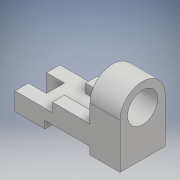
# Autodesk Inventor part: трон
Saved by Autodesk Inventor 2018 (Build 220112000, 112)
## iProperties
Created: 2020-04-15
Part Number: трон
Material: Типовые
Document SubType Name: Modeling
Designer: 2000
Density: 1 g/cm^3
Appearance: По умолчанию
Author: 2000
Autodesk Inventor part; units mm, degrees
ref_plane "YZ Plane" through (0, 0, 0) normal (1, 0, 0) x (0, 1, 0)
ref_plane "XZ Plane" through (0, 0, 0) normal (0, 1, 0) x (-1, 0, 0)
ref_plane "XY Plane" through (0, 0, 0) normal (0, 0, 1) x (1, 0, 0)
sketch "Эскиз1" plane through (0, 0, 0) normal (0, 0, 1) x (1, 0, 0)
  line L0 (-35, 15) -> (35, 15)
  line L1 (35, 15) -> (35, -15)
  line L2 (35, -15) -> (-35, -15)
  line L3 (-35, -15) -> (-35, 15)
  point P0 (0, 0)
  dimension "d0" = 70
  dimension "d1" = 30
  dimension "d2" = 15
  dimension "d3" = 35
  constraints: 8 end point, 2 parallel, 1 horizontal, 1 perpendicular
  measures "d0" distance of L0.start L0.end
  measures "d1" distance of L0.end L1.end
  measures "d2" distance from line of L0 point (0, 0)
  measures "d3" distance from line of L1 point (0, 0)
extrude "Выдавливание1" add sketch "Эскиз1" along normal blind 12
sketch "Эскиз2" plane through (0, 0, 12) normal (0, 0, 1) x (1, 0, 0)
  line L0 (-35, 6) -> (-23, 6)
  line L1 (-23, 6) -> (-23, -6)
  line L2 (-23, -6) -> (-35, -6)
  line L3 (-35, -6) -> (-35, 6)
  point P0 (0, 0)
  dimension "d6" = 6
  dimension "d7" = 6
  dimension "d8" = 12
  dimension "d9" = 35
  constraints: 8 end point, 2 parallel, 1 horizontal, 1 perpendicular
  measures "d6" distance from line of L0 point (0, 0)
  measures "d7" vertical distance of L1.end point (0, 0)
  measures "d8" distance between parallel lines of L1 L3
  measures "d9" distance from line of L3 point (0, 0)
extrude "Выдавливание2" cut sketch "Эскиз2" against normal blind 12
sketch "Эскиз3" plane through (-35, -15, 0) normal (0, -1, 0) x (1, 0, 0)
  line L0 (70, 0) -> (0, 0) projected
  line L1 (20, 0) -> (50, 0)
  line L2 (50, 0) -> (50, 5)
  line L3 (50, 5) -> (20, 5)
  line L4 (20, 5) -> (20, 0)
  point P0 (35, 0)
  dimension "d12" = 30
  dimension "d13" = 5
  dimension "d14" = 20
  constraints: 8 end point, 2 parallel, 1 horizontal, 1 perpendicular, 1 point on line
  measures "d12" distance of L2.end L3.end
  measures "d13" distance from line of point (35, 0) L3
  measures "d14" distance from line of L0.end L4
extrude "Выдавливание3" cut sketch "Эскиз3" against normal blind 30
sketch "Эскиз4" plane through (0, 0, 12) normal (0, 0, 1) x (1, 0, 0)
  line L0 (-10, 15) -> (15, 15)
  line L1 (15, 15) -> (15, 7)
  line L2 (15, 7) -> (-10, 7)
  line L3 (-10, 7) -> (-10, 15)
  line L4 (15, -15) -> (-10, -15)
  line L5 (-10, -15) -> (-10, -7)
  line L6 (-10, -7) -> (15, -7)
  line L7 (15, -7) -> (15, -15)
  line L8 (35, -15) -> (35, 15) projected
  line L9 (-35, 15) -> (-35, 6) projected
  line L10 (-35, -6) -> (-35, -15) projected
  line L11 (-35, 6) -> (-23, 6) projected
  line L12 (-23, 6) -> (-23, -6) projected
  line L13 (-23, -6) -> (-35, -6) projected
  line L14 (-35, -6) -> (-35, -15) projected
  line L15 (-35, -15) -> (35, -15) projected
  line L16 (35, -15) -> (35, 15) projected
  line L17 (35, 15) -> (-35, 15) projected
  line L18 (-35, 15) -> (-35, 6) projected
  point P0 (0, 0)
  dimension "d17" = 20
  dimension "d18" = 20
  dimension "d19" = 25
  dimension "d20" = 25
  dimension "d21" = 14
  dimension "d22" = 8
  dimension "d23" = 8
  dimension "d24" = 7
  constraints: 16 end point, 4 parallel, 2 horizontal, 2 perpendicular
  measures "d17" distance between parallel lines of L8 L7
  measures "d18" distance between parallel lines of L8 L1
  measures "d19" distance between parallel lines of L9 L3
  measures "d20" distance between parallel lines of L10 L5
  measures "d21" distance between parallel lines of L6 L2
  measures "d22" distance between parallel lines of L6 L4
  measures "d23" distance between parallel lines of L2 L0
  measures "d24" vertical distance of point (0, 0) L5.end
extrude "Выдавливание4" add sketch "Эскиз4" along normal blind 6 contours L0 L1 L2 L3 | L4 L5 L6 L7
sketch "Эскиз5" plane through (0, 0, 12) normal (0, 0, 1) x (1, 0, 0)
  line L0 (15, 15) -> (35, 15)
  line L1 (35, 15) -> (35, -15)
  line L2 (35, -15) -> (15, -15)
  line L3 (15, -15) -> (15, 15)
  point P0 (0, 0)
  constraints: 8 end point, 2 parallel, 1 horizontal, 1 perpendicular
extrude "Выдавливание5" add sketch "Эскиз5" along normal blind 18
sketch "Эскиз6" plane through (15, -7, 12) normal (-1, 0, 0) x (0, 0, 1)
  circle A0 centre (18, 7) radius 15
  point P0 (-12, 7)
  point P1 (18, 22)
  point P2 (18, -8)
  dimension "d29" = 30
  constraints: 2 point on circle, 1 centre point
  measures "d29" diameter of A0
extrude "Выдавливание6" add sketch "Эскиз6" against normal blind 20
sketch "Эскиз7" plane through (15, -7, 12) normal (-1, 0, 0) x (0, 0, 1)
  line L0 (0, 14) -> (6, 14) projected
  line L1 (0, 0) -> (0, 14) projected
  line L2 (0, 0) -> (6, 0) projected
  line L3 (6, -8) -> (6, 0) projected
  line L4 (6, -8) -> (18, -8) projected
  arc A0 (18, -8) -> (18, 22) centre (18, 7) ccw projected
  line L5 (6, 22) -> (18, 22) projected
  line L6 (6, 14) -> (6, 22) projected
  point P0 (-12, 7)
hole "Отверстие1" at (15, 0, 30) direction (1, 0, 0) diameter 20 depth 20 tip angle 118
